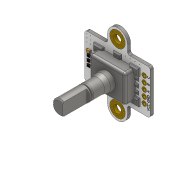
# Autodesk Inventor part: Rotary_Encoder_EC11
Saved by Autodesk Inventor 2017 (Build 210142000, 142)
## iProperties
Created: 2018-03-10
Part Number: Rotary_Encoder_EC11
Material: Generic
Document SubType Name: Modeling
Designer: Juan Carlos Botero
Density: 1 g/cm^3
Appearance: Stainless - Brushed
Author: Juan Carlos Botero
Autodesk Inventor part; units mm, degrees
ref_plane "YZ Plane" through (0, 0, 0) normal (1, 0, 0) x (0, 1, 0)
ref_plane "XZ Plane" through (0, 0, 0) normal (0, 1, 0) x (-1, 0, 0)
ref_plane "XY Plane" through (0, 0, 0) normal (0, 0, 1) x (1, 0, 0)
sketch "Sketch1" plane through (0, 0, 0) normal (0, 1, 0) x (-1, 0, 0)
  line L0 (13.715, 9.205) -> (13.715, -9.205)
  line L1 (-13.715, -9.205) -> (-13.715, 9.205)
  line L2 (-13.715, 9.205) -> (13.715, -9.205) construction
  line L3 (13.715, 9.205) -> (-13.715, -9.205) construction
  arc A0 (4.15, 12.7) -> (-4.15, 12.7) centre (0, 12.7) ccw
  arc A1 (-4.15, -12.7) -> (4.15, -12.7) centre (0, -12.7) ccw
  line L4 (0, 12.7) -> (0, -12.7) construction
  line L5 (4.15, 12.7) -> (4.15, 9.205)
  line L6 (4.15, -9.205) -> (4.15, -12.7)
  line L7 (-13.715, 9.205) -> (-4.15, 9.205)
  line L8 (4.15, 9.205) -> (13.715, 9.205)
  line L9 (13.715, -9.205) -> (4.15, -9.205)
  line L10 (-4.15, -9.205) -> (-13.715, -9.205)
  line L11 (-4.15, -12.7) -> (-4.15, -9.205)
  line L12 (-4.15, 9.205) -> (-4.15, 12.7)
  circle A2 centre (0, 12.7) radius 1.6
  circle A3 centre (0, -12.7) radius 1.6
  point P0 (0, 0)
  point P1 (0, 0)
  dimension "d0" = 27.43
  dimension "d1" = 18.41
  dimension "d2" = 25.4
  dimension "d3" = 8.3
  dimension "d4" = 3.2
  constraints: 26 end point, 5 parallel, 4 centre point, 4 midpoint, 4 point on circle, 4 tangent, 2 coincident, 2 equal radius, 2 horizontal, 2 perpendicular, 1 vertical
  measures "d0" distance of L0.end L1.start
  measures "d1" distance of L0.start L0.end
  measures "d2" distance of L4.start L4.end
  measures "d3" diameter of A1
  measures "d4" diameter of A2
extrude "Extrusion1" add sketch "Sketch1" along normal mid plane 1.32
fillet "Fillet1" radius 1 8 edges at (4.15, 0, 9.205) (-4.15, 0, 9.205) (-13.715, 0, 9.205) (-13.715, 0, -9.205) (-4.15, 0, -9.205) (4.15, 0, -9.205) (13.715, 0, -9.205) (13.715, 0, 9.205)
sketch "Sketch2" plane through (0, 0.66, 0) normal (0, 1, 0) x (1, 0, 0)
  arc A0 (12.715, -9.205) -> (13.715, -8.205) centre (12.715, -8.205) ccw projected
  line L0 (13.715, -8.205) -> (13.715, 8.205) projected
  arc A1 (13.715, 8.205) -> (12.715, 9.205) centre (12.715, 8.205) ccw projected
  line L1 (12.715, 9.205) -> (5.15, 9.205) projected
  arc A2 (4.15, 10.205) -> (5.15, 9.205) centre (5.15, 10.205) ccw projected
  line L2 (4.15, 10.205) -> (4.15, 12.7) projected
  arc A3 (4.15, 12.7) -> (-4.15, 12.7) centre (0, 12.7) ccw projected
  line L3 (-4.15, 12.7) -> (-4.15, 10.205) projected
  arc A4 (-5.15, 9.205) -> (-4.15, 10.205) centre (-5.15, 10.205) ccw projected
  line L4 (-5.15, 9.205) -> (-12.715, 9.205) projected
  arc A5 (-12.715, 9.205) -> (-13.715, 8.205) centre (-12.715, 8.205) ccw projected
  line L5 (-13.715, 8.205) -> (-13.715, -8.205) projected
  arc A6 (-13.715, -8.205) -> (-12.715, -9.205) centre (-12.715, -8.205) ccw projected
  line L6 (-12.715, -9.205) -> (-5.15, -9.205) projected
  arc A7 (-4.15, -10.205) -> (-5.15, -9.205) centre (-5.15, -10.205) ccw projected
  line L7 (-4.15, -10.205) -> (-4.15, -12.7) projected
  arc A8 (-4.15, -12.7) -> (4.15, -12.7) centre (0, -12.7) ccw projected
  line L8 (4.15, -12.7) -> (4.15, -10.205) projected
  arc A9 (5.15, -9.205) -> (4.15, -10.205) centre (5.15, -10.205) ccw projected
  line L9 (5.15, -9.205) -> (12.715, -9.205) projected
  circle A10 centre (0, 12.7) radius 1.6 projected
  circle A11 centre (0, -12.7) radius 1.6 projected
  circle A12 centre (0, -12.7) radius 3.25
  circle A13 centre (0, 12.7) radius 3.25
  point P0 (0, 0)
  dimension "d8" = 6.5
  dimension "d9" = 6.5
  constraints: 2 centre point, 2 coincident
  measures "d8" diameter of A12
  measures "d9" diameter of A13
extrude "Extrusion2" add sketch "Sketch2" along normal blind 0.01 contours A12 | A13
mirror "Mirror1" about plane through (0, 0, 0) normal (0, 1, 0) of "Extrusion2"
sketch "Sketch3" plane through (0, 0.67, -12.7) normal (0, 1, 0) x (1, 0, 0)
  circle A0 centre (0, -25.4) radius 1.6 projected
  circle A1 centre (0, -25.4) radius 3.25 projected
  circle A2 centre (-2.5, -25.4) radius 0.25
  circle A3 centre (0, -25.4) radius 2.5 construction
  point P0 (0, -12.7)
  dimension "d12" = 5
  dimension "d13" = 0.5
  constraints: 1 centre point, 1 coincident, 1 horizontal alignment, 2 other
  measures "d13" diameter of A2
extrude "Extrusion3" cut sketch "Sketch3" against normal through all contours A2
pattern_circular "Circular Pattern1" count 8 over 360 about axis through (0, 0, 12.7) along (0, 1, 0) of "Extrusion3"
sketch "Sketch4" plane through (0, 0.67, -12.7) normal (0, 1, 0) x (1, 0, 0)
  circle A0 centre (0, 0) radius 1.6 projected
  circle A1 centre (0, 0) radius 3.25 projected
  circle A2 centre (0, 0) radius 2.5 construction
  circle A3 centre (-2.5, 0) radius 0.25
  point P0 (0, -12.7)
  dimension "d19" = 5
  dimension "d20" = 0.5
  constraints: 1 centre point, 1 coincident, 1 horizontal alignment, 2 other
  measures "d20" diameter of A3
extrude "Extrusion4" cut sketch "Sketch4" against normal through all contours A3
pattern_circular "Circular Pattern2" count 8 over 360 about axis through (0, 0, -12.7) along (0, 1, 0) of "Extrusion4"
sketch "Sketch5" plane through (0, -0.66, 0) normal (0, -1, 0) x (1, 0, 0)
  line L0 (7.5, -6) -> (-7.5, -6)
  line L1 (-7.5, -6) -> (-7.5, 6)
  line L2 (-7.5, 6) -> (7.5, 6)
  line L3 (7.5, 6) -> (7.5, -6)
  line L4 (7.5, -6) -> (-7.5, 6) construction
  line L5 (-7.5, -6) -> (7.5, 6) construction
  point P0 (0, 0)
  dimension "d26" = 15
  dimension "d27" = 12
  constraints: 12 end point, 2 midpoint, 2 parallel, 1 horizontal, 1 perpendicular
  measures "d26" distance of L1.end L2.end
  measures "d27" distance of L0.end L1.end
extrude "Extrusion5" add sketch "Sketch5" along normal blind 4.4
sketch "Sketch6" plane through (0, -5.06, 0) normal (0, -1, 0) x (1, 0, 0)
  circle A0 centre (0, 0) radius 3.475
  dimension "d30" = 6.95
  constraints: 1 centre point, 1 coincident
  measures "d30" diameter of A0
extrude "Extrusion6" add sketch "Sketch6" along normal blind 2
sketch "Sketch7" plane through (0, -7.06, 0) normal (0, -1, 0) x (1, 0, 0)
  circle A0 centre (0, 0) radius 3.475 projected
extrude "Extrusion7" add sketch "Sketch7" along normal blind 2 draft -13
sketch "Sketch8" plane through (0, -9.06, 0) normal (0, -1, 0) x (1, 0, 0)
  circle A0 centre (0, 0) radius 3.0133 projected
extrude "Extrusion8" add sketch "Sketch8" along normal blind 5
fillet "Fillet2" radius 0.5 1 edges at (-3.0133, -14.06, 0)
sketch "Sketch9" plane through (0, -14.06, 0) normal (0, -1, 0) x (1, 0, 0)
  circle A0 centre (0, 0) radius 1.5
  dimension "d38" = 3
  constraints: 1 centre point, 1 coincident
  measures "d38" diameter of A0
extrude "Extrusion9" add sketch "Sketch9" along normal blind 0.5
sketch "Sketch10" plane through (0, -14.56, 0) normal (0, -1, 0) x (1, 0, 0)
  circle A0 centre (0, 0) radius 3.0133 projected
  circle A1 centre (0, 0) radius 3.0133 projected
extrude "Extrusion10" add sketch "Sketch10" along normal blind 10.5
chamfer "Chamfer1" distance 0.5 angle 45 1 edges at (-3.0133, -25.06, 0)
sketch "Sketch11" plane through (0, -25.06, 0) normal (0, -1, 0) x (1, 0, 0)
  line L0 (1.4867, 2.6209) -> (3.0133, 2.6209)
  line L1 (3.0133, 2.6209) -> (3.0133, -2.6209)
  line L2 (3.0133, -2.6209) -> (1.4867, -2.6209)
  line L3 (1.4867, -2.6209) -> (1.4867, 2.6209)
  circle A0 centre (0, 0) radius 3.0133 projected
  circle A1 centre (0, 0) radius 3.0133 projected
  line L4 (1.4867, 0) -> (-3.0133, 0)
  point P0 (3.0133, 0)
  dimension "d46" = 4.5
  constraints: 10 end point, 3 point on circle, 2 horizontal, 2 midpoint, 2 parallel, 1 horizontal alignment, 1 perpendicular, 1 point on line, 1 other
  measures "d46" distance of L4.start L4.end
extrude "Extrusion11" cut sketch "Sketch11" against normal blind 10 contours A0 L3 | L0 L1 A0 | L1 L2 A0
sketch "Sketch12" plane through (0, -0.66, 0) normal (0, -1, 0) x (1, 0, 0)
  circle A0 centre (11.215, -5.08) radius 0.5
  circle A1 centre (11.215, -2.54) radius 0.5
  circle A2 centre (11.215, 0) radius 0.5
  circle A3 centre (11.215, 2.54) radius 0.5
  circle A4 centre (11.215, 5.08) radius 0.5
  line L0 (13.715, -8.205) -> (13.715, 8.205) projected
  point P0 (0, 0)
  dimension "d49" = 2.54
  dimension "d50" = 2.54
  dimension "d51" = 2.54
  dimension "d52" = 2.54
  dimension "d53" = 1
  dimension "d54" = 2.5
  constraints: 5 centre point, 4 equal radius, 4 vertical alignment, 1 horizontal alignment
  measures "d49" distance of A1.centre A0.centre
  measures "d50" distance of A1.centre A2.centre
  measures "d51" distance of A2.centre A3.centre
  measures "d52" distance of A3.centre A4.centre
  measures "d53" diameter of A0
  measures "d54" distance from line of L0 A1.centre
extrude "Extrusion12" cut sketch "Sketch12" against normal through all
sketch "Sketch13" plane through (0, -0.66, 0) normal (0, -1, 0) x (1, 0, 0)
  circle A0 centre (11.215, 2.54) radius 0.5 projected
  circle A1 centre (11.215, -2.54) radius 0.5 projected
  circle A2 centre (11.215, -5.08) radius 0.5 projected
  circle A3 centre (11.215, 0) radius 0.5 projected
  circle A4 centre (11.215, 5.08) radius 0.5 projected
  line L0 (-7.5, -6) -> (-7.5, 6) projected
  line L1 (-7.5, 6) -> (7.5, 6) projected
  line L2 (7.5, 6) -> (7.5, -6) projected
  line L3 (7.5, -6) -> (-7.5, -6) projected
  circle A5 centre (0, 12.7) radius 3.25 projected
  circle A6 centre (0, -12.7) radius 3.25 projected
  arc A7 (13.715, 8.205) -> (12.715, 9.205) centre (12.715, 8.205) ccw projected
  line L4 (12.715, 9.205) -> (5.15, 9.205) projected
  arc A8 (4.15, 10.205) -> (5.15, 9.205) centre (5.15, 10.205) ccw projected
  line L5 (4.15, 10.205) -> (4.15, 12.7) projected
  arc A9 (4.15, 12.7) -> (-4.15, 12.7) centre (0, 12.7) ccw projected
  line L6 (-4.15, 12.7) -> (-4.15, 10.205) projected
  arc A10 (-5.15, 9.205) -> (-4.15, 10.205) centre (-5.15, 10.205) ccw projected
  line L7 (-5.15, 9.205) -> (-12.715, 9.205) projected
  arc A11 (-12.715, 9.205) -> (-13.715, 8.205) centre (-12.715, 8.205) ccw projected
  line L8 (-13.715, 8.205) -> (-13.715, -8.205) projected
  arc A12 (-13.715, -8.205) -> (-12.715, -9.205) centre (-12.715, -8.205) ccw projected
  line L9 (-12.715, -9.205) -> (-5.15, -9.205) projected
  arc A13 (-4.15, -10.205) -> (-5.15, -9.205) centre (-5.15, -10.205) ccw projected
  line L10 (-4.15, -10.205) -> (-4.15, -12.7) projected
  arc A14 (-4.15, -12.7) -> (4.15, -12.7) centre (0, -12.7) ccw projected
  line L11 (4.15, -12.7) -> (4.15, -10.205) projected
  arc A15 (5.15, -9.205) -> (4.15, -10.205) centre (5.15, -10.205) ccw projected
  line L12 (5.15, -9.205) -> (12.715, -9.205) projected
  arc A16 (12.715, -9.205) -> (13.715, -8.205) centre (12.715, -8.205) ccw projected
  line L13 (13.715, -8.205) -> (13.715, 8.205) projected
  circle A17 centre (11.215, -5.08) radius 1
  circle A18 centre (11.215, -2.54) radius 1
  circle A19 centre (11.215, 0) radius 1
  circle A20 centre (11.215, 2.54) radius 1
  circle A21 centre (11.215, 5.08) radius 1
  point P0 (0, 0)
  dimension "d57" = 0.5
  constraints: 5 centre point, 4 equal radius
  measures "d57" radial gap between concentric circles of A2 A17
extrude "Extrusion13" add sketch "Sketch13" along normal blind 0.01 contours A17 | A18 | A19 | A20 | A21
mirror "Mirror2" about plane through (0, 0, 0) normal (0, 1, 0) of "Extrusion13"
fillet "Fillet3" radius 1 8 edges at (0, -5.06, -6) (7.5, -5.06, 0) (7.5, -2.86, -6) (7.5, -2.86, 6) (0, -5.06, 6) (-7.5, -2.86, 6) (-7.5, -5.06, 0) (-7.5, -2.86, -6)
sketch "Sketch14" plane through (0, -0.66, 0) normal (0, -1, 0) x (1, 0, 0)
  line L0 (12.4092, -6.8272) -> (12.4092, 6.4026) construction
  line L1 (12.4092, 6.4026) -> (14.0609, 6.4026) construction
  line L2 (14.0609, 6.4026) -> (14.0609, -6.8272) construction
  line L3 (14.0609, -6.8272) -> (12.4092, -6.8272) construction
  line L4 (12.4271, -6.0006) -> (13.4271, -6.345)
  line L5 (13.4271, -6.345) -> (13.4271, -6.4885)
  line L6 (13.4271, -6.4885) -> (12.4271, -6.8329)
  line L7 (12.4271, -6.8329) -> (12.4271, -6.6903)
  line L8 (12.4271, -6.6903) -> (13.2577, -6.4131)
  line L9 (13.2577, -6.4131) -> (12.4271, -6.136)
  line L10 (12.4271, -6.136) -> (12.4271, -6.0006)
  spline S0 degree 2 poles (13.4449, -5.5144) (13.4449, -5.6117) (13.3793, -5.7762) (13.3136, -5.8361) knots 0 0 0 1 2 2 2
  spline S1 degree 2 poles (13.3136, -5.8361) (13.2488, -5.8961) (13.0543, -5.9617) (12.9279, -5.9617) knots 0 0 0 1 2 2 2
  spline S2 degree 2 poles (12.9279, -5.9617) (12.8023, -5.9617) (12.6159, -5.8977) (12.547, -5.8369) knots 0 0 0 1 2 2 2
  spline S3 degree 2 poles (12.547, -5.8369) (12.4797, -5.777) (12.4092, -5.6133) (12.4092, -5.512) knots 0 0 0 1 2 2 2
  spline S4 degree 2 poles (12.4092, -5.512) (12.4092, -5.4617) (12.4238, -5.3734) (12.4352, -5.3361) knots 0 0 0 1 2 2 2
  spline S5 degree 2 poles (12.4352, -5.3361) (12.4457, -5.3037) (12.4757, -5.2365) (12.4935, -5.2032) knots 0 0 0 1 2 2 2
  line L11 (12.4935, -5.2032) -> (12.654, -5.2032)
  line L12 (12.654, -5.2032) -> (12.654, -5.2138)
  spline S6 degree 2 poles (12.654, -5.2138) (12.6378, -5.2316) (12.5924, -5.2867) (12.5705, -5.3264) knots 0 0 0 1 2 2 2
  spline S7 degree 2 poles (12.5705, -5.3264) (12.5494, -5.3645) (12.5227, -5.4544) (12.5227, -5.5128) knots 0 0 0 1 2 2 2
  spline S8 degree 2 poles (12.5227, -5.5128) (12.5227, -5.5768) (12.5754, -5.6911) (12.6256, -5.734) knots 0 0 0 1 2 2 2
  spline S9 degree 2 poles (12.6256, -5.734) (12.6767, -5.7762) (12.8314, -5.8232) (12.9279, -5.8232) knots 0 0 0 1 2 2 2
  spline S10 degree 2 poles (12.9279, -5.8232) (13.0308, -5.8232) (13.1791, -5.7737) (13.2301, -5.7308) knots 0 0 0 1 2 2 2
  spline S11 degree 2 poles (13.2301, -5.7308) (13.2796, -5.6886) (13.3298, -5.576) (13.3298, -5.5128) knots 0 0 0 1 2 2 2
  spline S12 degree 2 poles (13.3298, -5.5128) (13.3298, -5.4553) (13.3015, -5.3572) (13.2804, -5.3191) knots 0 0 0 1 2 2 2
  spline S13 degree 2 poles (13.2804, -5.3191) (13.2593, -5.2827) (13.2156, -5.2284) (13.2002, -5.213) knots 0 0 0 1 2 2 2
  line L13 (13.2002, -5.213) -> (13.2002, -5.2032)
  line L14 (13.2002, -5.2032) -> (13.359, -5.2032)
  spline S14 degree 2 poles (13.359, -5.2032) (13.3744, -5.2365) (13.4028, -5.2948) (13.4157, -5.3361) knots 0 0 0 1 2 2 2
  spline S15 degree 2 poles (13.4157, -5.3361) (13.4303, -5.3799) (13.4449, -5.4544) (13.4449, -5.5144) knots 0 0 0 1 2 2 2
  spline S16 degree 2 poles (13.4449, -4.6886) (13.4449, -4.7859) (13.3793, -4.9504) (13.3136, -5.0104) knots 0 0 0 1 2 2 2
  spline S17 degree 2 poles (13.3136, -5.0104) (13.2488, -5.0703) (13.0543, -5.136) (12.9279, -5.136) knots 0 0 0 1 2 2 2
  spline S18 degree 2 poles (12.9279, -5.136) (12.8023, -5.136) (12.6159, -5.072) (12.547, -5.0112) knots 0 0 0 1 2 2 2
  spline S19 degree 2 poles (12.547, -5.0112) (12.4797, -4.9512) (12.4092, -4.7875) (12.4092, -4.6862) knots 0 0 0 1 2 2 2
  spline S20 degree 2 poles (12.4092, -4.6862) (12.4092, -4.636) (12.4238, -4.5476) (12.4352, -4.5104) knots 0 0 0 1 2 2 2
  spline S21 degree 2 poles (12.4352, -4.5104) (12.4457, -4.478) (12.4757, -4.4107) (12.4935, -4.3775) knots 0 0 0 1 2 2 2
  line L15 (12.4935, -4.3775) -> (12.654, -4.3775)
  line L16 (12.654, -4.3775) -> (12.654, -4.388)
  spline S22 degree 2 poles (12.654, -4.388) (12.6378, -4.4058) (12.5924, -4.4609) (12.5705, -4.5006) knots 0 0 0 1 2 2 2
  spline S23 degree 2 poles (12.5705, -4.5006) (12.5494, -4.5387) (12.5227, -4.6287) (12.5227, -4.687) knots 0 0 0 1 2 2 2
  spline S24 degree 2 poles (12.5227, -4.687) (12.5227, -4.751) (12.5754, -4.8653) (12.6256, -4.9083) knots 0 0 0 1 2 2 2
  spline S25 degree 2 poles (12.6256, -4.9083) (12.6767, -4.9504) (12.8314, -4.9974) (12.9279, -4.9974) knots 0 0 0 1 2 2 2
  spline S26 degree 2 poles (12.9279, -4.9974) (13.0308, -4.9974) (13.1791, -4.948) (13.2301, -4.905) knots 0 0 0 1 2 2 2
  spline S27 degree 2 poles (13.2301, -4.905) (13.2796, -4.8629) (13.3298, -4.7502) (13.3298, -4.687) knots 0 0 0 1 2 2 2
  spline S28 degree 2 poles (13.3298, -4.687) (13.3298, -4.6295) (13.3015, -4.5314) (13.2804, -4.4933) knots 0 0 0 1 2 2 2
  spline S29 degree 2 poles (13.2804, -4.4933) (13.2593, -4.4569) (13.2156, -4.4026) (13.2002, -4.3872) knots 0 0 0 1 2 2 2
  line L17 (13.2002, -4.3872) -> (13.2002, -4.3775)
  line L18 (13.2002, -4.3775) -> (13.359, -4.3775)
  spline S30 degree 2 poles (13.359, -4.3775) (13.3744, -4.4107) (13.4028, -4.469) (13.4157, -4.5104) knots 0 0 0 1 2 2 2
  spline S31 degree 2 poles (13.4157, -4.5104) (13.4303, -4.5541) (13.4449, -4.6287) (13.4449, -4.6886) knots 0 0 0 1 2 2 2
  spline S32 degree 2 poles (13.4465, -3.405) (13.4465, -3.5112) (13.3817, -3.687) (13.316, -3.7502) knots 0 0 0 1 2 2 2
  spline S33 degree 2 poles (13.316, -3.7502) (13.2496, -3.8134) (13.0535, -3.8807) (12.9263, -3.8807) knots 0 0 0 1 2 2 2
  spline S34 degree 2 poles (12.9263, -3.8807) (12.8055, -3.8807) (12.6143, -3.8126) (12.5462, -3.7494) knots 0 0 0 1 2 2 2
  spline S35 degree 2 poles (12.5462, -3.7494) (12.4806, -3.6886) (12.4092, -3.5104) (12.4092, -3.4042) knots 0 0 0 1 2 2 2
  spline S36 degree 2 poles (12.4092, -3.4042) (12.4092, -3.3532) (12.4238, -3.2608) (12.4368, -3.2186) knots 0 0 0 1 2 2 2
  spline S37 degree 2 poles (12.4368, -3.2186) (12.4465, -3.1846) (12.4822, -3.1019) (12.4951, -3.0768) knots 0 0 0 1 2 2 2
  line L19 (12.4951, -3.0768) -> (12.6556, -3.0768)
  line L20 (12.6556, -3.0768) -> (12.6556, -3.0882)
  spline S38 degree 2 poles (12.6556, -3.0882) (12.6337, -3.1133) (12.594, -3.166) (12.5713, -3.2146) knots 0 0 0 1 2 2 2
  spline S39 degree 2 poles (12.5713, -3.2146) (12.5511, -3.2551) (12.5243, -3.3596) (12.5243, -3.4196) knots 0 0 0 1 2 2 2
  spline S40 degree 2 poles (12.5243, -3.4196) (12.5243, -3.5638) (12.7415, -3.7421) (12.9222, -3.7421) knots 0 0 0 1 2 2 2
  spline S41 degree 2 poles (12.9222, -3.7421) (13.0227, -3.7421) (13.1734, -3.6951) (13.2253, -3.6506) knots 0 0 0 1 2 2 2
  spline S42 degree 2 poles (13.2253, -3.6506) (13.2771, -3.6076) (13.3314, -3.4861) (13.3314, -3.4099) knots 0 0 0 1 2 2 2
  spline S43 degree 2 poles (13.3314, -3.4099) (13.3314, -3.354) (13.3152, -3.2421) (13.299, -3.204) knots 0 0 0 1 2 2 2
  line L21 (13.299, -3.204) -> (13.0405, -3.204)
  line L22 (13.0405, -3.204) -> (13.0405, -3.4358)
  line L23 (13.0405, -3.4358) -> (12.9238, -3.4358)
  line L24 (12.9238, -3.4358) -> (12.9238, -3.0728)
  line L25 (12.9238, -3.0728) -> (13.3606, -3.0728)
  spline S44 degree 2 poles (13.3606, -3.0728) (13.372, -3.0979) (13.4068, -3.1838) (13.4173, -3.2203) knots 0 0 0 1 2 2 2
  spline S45 degree 2 poles (13.4173, -3.2203) (13.4319, -3.2697) (13.4465, -3.3491) (13.4465, -3.405) knots 0 0 0 1 2 2 2
  line L26 (13.4271, -2.1903) -> (13.4271, -2.3394)
  line L27 (13.4271, -2.3394) -> (12.5648, -2.7818)
  line L28 (12.5648, -2.7818) -> (13.4271, -2.7818)
  line L29 (13.4271, -2.7818) -> (13.4271, -2.9058)
  line L30 (13.4271, -2.9058) -> (12.4271, -2.9058)
  line L31 (12.4271, -2.9058) -> (12.4271, -2.717)
  line L32 (12.4271, -2.717) -> (13.2188, -2.3143)
  line L33 (13.2188, -2.3143) -> (12.4271, -2.3143)
  line L34 (12.4271, -2.3143) -> (12.4271, -2.1903)
  line L35 (12.4271, -2.1903) -> (13.4271, -2.1903)
  spline S46 degree 2 poles (12.9279, -1.1992) (13.0648, -1.1992) (13.2853, -1.3102) (13.3468, -1.4034) knots 0 0 0 1 2 2 2
  spline S47 degree 2 poles (13.3468, -1.4034) (13.3947, -1.4796) (13.4271, -1.636) (13.4271, -1.7575) knots 0 0 0 1 2 2 2
  line L36 (13.4271, -1.7575) -> (13.4271, -1.9877)
  line L37 (13.4271, -1.9877) -> (12.4271, -1.9877)
  line L38 (12.4271, -1.9877) -> (12.4271, -1.76)
  spline S48 degree 2 poles (12.4271, -1.76) (12.4271, -1.619) (12.4692, -1.4585) (12.5065, -1.4018) knots 0 0 0 1 2 2 2
  spline S49 degree 2 poles (12.5065, -1.4018) (12.5705, -1.3053) (12.782, -1.1992) (12.9279, -1.1992) knots 0 0 0 1 2 2 2
  spline S50 degree 2 poles (12.9263, -1.3378) (12.8112, -1.3378) (12.6483, -1.4139) (12.6021, -1.4893) knots 0 0 0 1 2 2 2
  spline S51 degree 2 poles (12.6021, -1.4893) (12.5705, -1.5428) (12.5421, -1.6635) (12.5421, -1.7535) knots 0 0 0 1 2 2 2
  line L39 (12.5421, -1.7535) -> (12.5421, -1.8548)
  line L40 (12.5421, -1.8548) -> (13.312, -1.8548)
  line L41 (13.312, -1.8548) -> (13.312, -1.7535)
  spline S52 degree 2 poles (13.312, -1.7535) (13.312, -1.6651) (13.2836, -1.5314) (13.2455, -1.4771) knots 0 0 0 1 2 2 2
  spline S53 degree 2 poles (13.2455, -1.4771) (13.1985, -1.4074) (13.043, -1.3378) (12.9263, -1.3378) knots 0 0 0 1 2 2 2
  line L42 (13.4271, -0.3037) -> (12.4271, 0.0334)
  line L43 (12.4271, 0.0334) -> (12.4271, 0.1971)
  line L44 (12.4271, 0.1971) -> (13.4271, 0.5342)
  line L45 (13.4271, 0.5342) -> (13.4271, 0.394)
  line L46 (13.4271, 0.394) -> (13.1475, 0.3032)
  line L47 (13.1475, 0.3032) -> (13.1475, -0.0784)
  line L48 (13.1475, -0.0784) -> (13.4271, -0.1692)
  line L49 (13.4271, -0.1692) -> (13.4271, -0.3037)
  line L50 (13.034, 0.2668) -> (12.5632, 0.112)
  line L51 (12.5632, 0.112) -> (13.034, -0.042)
  line L52 (13.034, -0.042) -> (13.034, 0.2668)
  spline S54 degree 2 poles (13.1199, 3.0253) (13.1945, 3.0253) (13.3088, 2.9686) (13.346, 2.9216) knots 0 0 0 1 2 2 2
  spline S55 degree 2 poles (13.346, 2.9216) (13.3898, 2.8648) (13.4271, 2.736) (13.4271, 2.6339) knots 0 0 0 1 2 2 2
  line L53 (13.4271, 2.6339) -> (13.4271, 2.347)
  line L54 (13.4271, 2.347) -> (12.4271, 2.347)
  line L55 (12.4271, 2.347) -> (12.4271, 2.612)
  spline S56 degree 2 poles (12.4271, 2.612) (12.4271, 2.719) (12.4408, 2.8259) (12.4676, 2.8746) knots 0 0 0 1 2 2 2
  spline S57 degree 2 poles (12.4676, 2.8746) (12.4959, 2.9289) (12.5891, 2.9783) (12.6524, 2.9783) knots 0 0 0 1 2 2 2
  spline S58 degree 2 poles (12.6524, 2.9783) (12.7229, 2.9783) (12.8347, 2.9037) (12.8663, 2.8381) knots 0 0 0 1 2 2 2
  line L56 (12.8663, 2.8381) -> (12.8712, 2.8381)
  spline S59 degree 2 poles (12.8712, 2.8381) (12.8955, 2.9272) (13.0243, 3.0253) (13.1199, 3.0253) knots 0 0 0 1 2 2 2
  spline S60 degree 2 poles (13.1256, 2.8867) (13.0689, 2.8867) (12.9959, 2.8543) (12.97, 2.8057) knots 0 0 0 1 2 2 2
  spline S61 degree 2 poles (12.97, 2.8057) (12.9538, 2.7741) (12.9441, 2.6995) (12.9441, 2.6306) knots 0 0 0 1 2 2 2
  line L57 (12.9441, 2.6306) -> (12.9441, 2.4799)
  line L58 (12.9441, 2.4799) -> (13.3136, 2.4799)
  line L59 (13.3136, 2.4799) -> (13.3136, 2.5877)
  spline S62 degree 2 poles (13.3136, 2.5877) (13.3136, 2.6752) (13.2974, 2.7757) (13.2715, 2.8146) knots 0 0 0 1 2 2 2
  spline S63 degree 2 poles (13.2715, 2.8146) (13.2447, 2.8519) (13.1783, 2.8867) (13.1256, 2.8867) knots 0 0 0 1 2 2 2
  spline S64 degree 2 poles (12.671, 2.8397) (12.6353, 2.8397) (12.5818, 2.8154) (12.5665, 2.7887) knots 0 0 0 1 2 2 2
  spline S65 degree 2 poles (12.5665, 2.7887) (12.5486, 2.7562) (12.5405, 2.6776) (12.5405, 2.6071) knots 0 0 0 1 2 2 2
  line L60 (12.5405, 2.6071) -> (12.5405, 2.4799)
  line L61 (12.5405, 2.4799) -> (12.8331, 2.4799)
  line L62 (12.8331, 2.4799) -> (12.8331, 2.6306)
  spline S66 degree 2 poles (12.8331, 2.6306) (12.8331, 2.693) (12.8201, 2.7522) (12.7998, 2.7838) knots 0 0 0 1 2 2 2
  spline S67 degree 2 poles (12.7998, 2.7838) (12.7804, 2.8146) (12.718, 2.8397) (12.671, 2.8397) knots 0 0 0 1 2 2 2
  spline S68 degree 2 poles (13.4449, 5.266) (13.4449, 5.1687) (13.3793, 5.0042) (13.3136, 4.9443) knots 0 0 0 1 2 2 2
  spline S69 degree 2 poles (13.3136, 4.9443) (13.2488, 4.8843) (13.0543, 4.8186) (12.9279, 4.8186) knots 0 0 0 1 2 2 2
  spline S70 degree 2 poles (12.9279, 4.8186) (12.8023, 4.8186) (12.6159, 4.8827) (12.547, 4.9434) knots 0 0 0 1 2 2 2
  spline S71 degree 2 poles (12.547, 4.9434) (12.4797, 5.0034) (12.4092, 5.1671) (12.4092, 5.2684) knots 0 0 0 1 2 2 2
  spline S72 degree 2 poles (12.4092, 5.2684) (12.4092, 5.3186) (12.4238, 5.407) (12.4352, 5.4443) knots 0 0 0 1 2 2 2
  spline S73 degree 2 poles (12.4352, 5.4443) (12.4457, 5.4767) (12.4757, 5.5439) (12.4935, 5.5772) knots 0 0 0 1 2 2 2
  line L63 (12.4935, 5.5772) -> (12.654, 5.5772)
  line L64 (12.654, 5.5772) -> (12.654, 5.5666)
  spline S74 degree 2 poles (12.654, 5.5666) (12.6378, 5.5488) (12.5924, 5.4937) (12.5705, 5.454) knots 0 0 0 1 2 2 2
  spline S75 degree 2 poles (12.5705, 5.454) (12.5494, 5.4159) (12.5227, 5.3259) (12.5227, 5.2676) knots 0 0 0 1 2 2 2
  spline S76 degree 2 poles (12.5227, 5.2676) (12.5227, 5.2036) (12.5754, 5.0893) (12.6256, 5.0464) knots 0 0 0 1 2 2 2
  spline S77 degree 2 poles (12.6256, 5.0464) (12.6767, 5.0042) (12.8314, 4.9572) (12.9279, 4.9572) knots 0 0 0 1 2 2 2
  spline S78 degree 2 poles (12.9279, 4.9572) (13.0308, 4.9572) (13.1791, 5.0067) (13.2301, 5.0496) knots 0 0 0 1 2 2 2
  spline S79 degree 2 poles (13.2301, 5.0496) (13.2796, 5.0917) (13.3298, 5.2044) (13.3298, 5.2676) knots 0 0 0 1 2 2 2
  spline S80 degree 2 poles (13.3298, 5.2676) (13.3298, 5.3251) (13.3015, 5.4232) (13.2804, 5.4613) knots 0 0 0 1 2 2 2
  spline S81 degree 2 poles (13.2804, 5.4613) (13.2593, 5.4977) (13.2156, 5.552) (13.2002, 5.5674) knots 0 0 0 1 2 2 2
  line L65 (13.2002, 5.5674) -> (13.2002, 5.5772)
  line L66 (13.2002, 5.5772) -> (13.359, 5.5772)
  spline S82 degree 2 poles (13.359, 5.5772) (13.3744, 5.5439) (13.4028, 5.4856) (13.4157, 5.4443) knots 0 0 0 1 2 2 2
  spline S83 degree 2 poles (13.4157, 5.4443) (13.4303, 5.4005) (13.4449, 5.3259) (13.4449, 5.266) knots 0 0 0 1 2 2 2
  point P0 (0, 0)
  constraints: 2 other
extrude "Extrusion14" add sketch "Sketch14" along normal blind 0.01
sketch "Sketch15" plane through (0, -0.66, 0) normal (0, -1, 0) x (1, 0, 0)
  line L0 (-1.75, 5.5) -> (1.75, 5.5)
  line L1 (1.75, 5.5) -> (1.75, 8)
  line L2 (1.75, 8) -> (-1.75, 8)
  line L3 (-1.75, 8) -> (-1.75, 5.5)
  line L4 (-1.75, 5.5) -> (1.75, 8) construction
  line L5 (1.75, 5.5) -> (-1.75, 8) construction
  line L6 (-1.75, -8) -> (1.75, -8)
  line L7 (1.75, -8) -> (1.75, -5.5)
  line L8 (1.75, -5.5) -> (-1.75, -5.5)
  line L9 (-1.75, -5.5) -> (-1.75, -8)
  line L10 (-1.75, -8) -> (1.75, -5.5) construction
  line L11 (1.75, -8) -> (-1.75, -5.5) construction
  line L12 (0, 6.75) -> (0, -6.75) construction
  line L13 (7, 1.75) -> (9, 1.75)
  line L14 (9, 1.75) -> (9, 3.25)
  line L15 (9, 3.25) -> (7, 3.25)
  line L16 (7, 3.25) -> (7, 1.75)
  line L17 (7, 1.75) -> (9, 3.25) construction
  line L18 (9, 1.75) -> (7, 3.25) construction
  line L19 (7, -0.75) -> (9, -0.75)
  line L20 (9, -0.75) -> (9, 0.75)
  line L21 (9, 0.75) -> (7, 0.75)
  line L22 (7, 0.75) -> (7, -0.75)
  line L23 (7, -0.75) -> (9, 0.75) construction
  line L24 (9, -0.75) -> (7, 0.75) construction
  line L25 (7, -3.25) -> (9, -3.25)
  line L26 (9, -3.25) -> (9, -1.75)
  line L27 (9, -1.75) -> (7, -1.75)
  line L28 (7, -1.75) -> (7, -3.25)
  line L29 (7, -3.25) -> (9, -1.75) construction
  line L30 (9, -3.25) -> (7, -1.75) construction
  line L31 (8, -2.5) -> (8, 2.5) construction
  line L32 (-9, 1.75) -> (-7, 1.75)
  line L33 (-7, 1.75) -> (-7, 3.25)
  line L34 (-7, 3.25) -> (-9, 3.25)
  line L35 (-9, 3.25) -> (-9, 1.75)
  line L36 (-9, 1.75) -> (-7, 3.25) construction
  line L37 (-7, 1.75) -> (-9, 3.25) construction
  line L38 (-9, -3.25) -> (-7, -3.25)
  line L39 (-7, -3.25) -> (-7, -1.75)
  line L40 (-7, -1.75) -> (-9, -1.75)
  line L41 (-9, -1.75) -> (-9, -3.25)
  line L42 (-9, -3.25) -> (-7, -1.75) construction
  line L43 (-7, -3.25) -> (-9, -1.75) construction
  line L44 (-8, 2.5) -> (8, -2.5) construction
  line L45 (-8, -2.5) -> (8, 2.5) construction
  point P0 (0, 0)
  point P1 (0, 0)
  point P2 (8, 2.5)
  point P3 (8, 0)
  point P4 (8, -2.5)
  point P5 (8, 2.5)
  point P6 (8, 0)
  point P7 (8, 0)
  point P8 (0, 0)
  dimension "d63" = 2.5
  dimension "d64" = 3.5
  dimension "d65" = 16
  dimension "d67" = 2
  dimension "d68" = 1.5
  dimension "d69" = 6.5
  dimension "d72" = 6.5
  dimension "d73" = 18
  constraints: 92 end point, 23 midpoint, 14 parallel, 11 equal length, 7 horizontal, 7 perpendicular, 3 point on line, 3 vertical alignment, 2 vertical, 1 coincident, 1 horizontal alignment
  measures "d63" distance of L2.end L0.start
  measures "d64" distance of L1.end L2.end
  measures "d65" distance between parallel lines of L6 L2
  measures "d67" distance of L14.end L15.end
  measures "d68" distance of L13.end L14.end
  measures "d69" distance between parallel lines of L25 L15
  measures "d72" distance between parallel lines of L38 L34
  measures "d73" distance between parallel lines of L26 L41
extrude "Extrusion15" add sketch "Sketch15" along normal blind 0.5
sketch "Sketch16" plane through (0, -0.66, 0) normal (0, -1, 0) x (1, 0, 0)
  line L0 (-9.5, 4) -> (-5.5, 4)
  line L1 (-5.5, 4) -> (-5.5, 7)
  line L2 (-5.5, 7) -> (-9.5, 7)
  line L3 (-9.5, 7) -> (-9.5, 4)
  line L4 (-9.5, 4) -> (-5.5, 7) construction
  line L5 (-5.5, 4) -> (-9.5, 7) construction
  line L6 (5.5, 4) -> (9.5, 4)
  line L7 (9.5, 4) -> (9.5, 7)
  line L8 (9.5, 7) -> (5.5, 7)
  line L9 (5.5, 7) -> (5.5, 4)
  line L10 (5.5, 4) -> (9.5, 7) construction
  line L11 (9.5, 4) -> (5.5, 7) construction
  line L12 (5.5, -7) -> (9.5, -7)
  line L13 (9.5, -7) -> (9.5, -4)
  line L14 (9.5, -4) -> (5.5, -4)
  line L15 (5.5, -4) -> (5.5, -7)
  line L16 (5.5, -7) -> (9.5, -4) construction
  line L17 (9.5, -7) -> (5.5, -4) construction
  line L18 (-9.5, -7) -> (-5.5, -7)
  line L19 (-5.5, -7) -> (-5.5, -4)
  line L20 (-5.5, -4) -> (-9.5, -4)
  line L21 (-9.5, -4) -> (-9.5, -7)
  line L22 (-9.5, -7) -> (-5.5, -4) construction
  line L23 (-5.5, -7) -> (-9.5, -4) construction
  line L24 (6.5, 6) -> (-6.5, 6) projected
  line L25 (-6.5, -6) -> (6.5, -6) projected
  line L26 (-7.5, 5) -> (-7.5, -5) projected
  line L27 (7.5, -5) -> (7.5, 5) projected
  point P0 (0, 0)
  point P1 (-7.5, 5.5)
  point P2 (7.5, 5.5)
  point P3 (7.5, -5.5)
  point P4 (-7.5, -5.5)
  point P5 (-7.5, 5.5)
  point P6 (7.5, 5.5)
  point P7 (-7.5, -5.5)
  point P8 (7.5, -5.5)
  point P9 (-7.5, 5.5)
  point P10 (-7.5, -5.5)
  point P11 (7.5, 5.5)
  point P12 (7.5, -5.5)
  dimension "d76" = 1
  dimension "d77" = 1
  dimension "d78" = 3
  dimension "d79" = 4
  dimension "d80" = 2
  dimension "d81" = 2
  constraints: 48 end point, 16 midpoint, 8 parallel, 6 equal length, 4 horizontal, 4 perpendicular, 2 horizontal alignment, 2 vertical alignment, 1 point on line
  measures "d76" distance between parallel lines of L24 L2
  measures "d77" distance between parallel lines of L25 L18
  measures "d78" distance of L2.end L0.start
  measures "d79" distance of L1.end L2.end
  measures "d80" distance between parallel lines of L3 L26
  measures "d81" distance between parallel lines of L7 L27
extrude "Extrusion16" add sketch "Sketch16" along normal blind 1 contours L3 L2 L1 L0 | L20 L19 L18 L21 | L9 L8 L7 L6 | L15 L14 L13 L12
sketch "Sketch17" plane through (0, -0.66, 0) normal (0, -1, 0) x (1, 0, 0)
  circle A0 centre (0, 2.5) radius 0.5
  circle A1 centre (0, -2) radius 0.6
  point P0 (0, 0)
  dimension "d84" = 1
  dimension "d85" = 1.2
  dimension "d86" = 2.5
  dimension "d87" = 2
  constraints: 2 centre point, 2 vertical alignment
  measures "d84" diameter of A0
  measures "d85" diameter of A1
  measures "d86" distance of point (0, 0) A0.centre
  measures "d87" distance of A1.centre point (0, 0)
extrude "Extrusion17" cut sketch "Sketch17" against normal through all
sketch "Sketch18" plane through (0, -0.66, -2) normal (0, 1, 0) x (1, 0, 0)
  circle A0 centre (0, -4.5) radius 0.5 projected
  circle A1 centre (0, 0) radius 0.6 projected
  circle A2 centre (11.215, -7.08) radius 1 projected
  circle A3 centre (11.215, -2) radius 1 projected
  circle A4 centre (11.215, 3.08) radius 1 projected
  circle A5 centre (11.215, 0.54) radius 1 projected
  circle A6 centre (11.215, -4.54) radius 1 projected
  circle A7 centre (0, -14.7) radius 3.25 projected
  circle A8 centre (0, 10.7) radius 3.25 projected
  arc A9 (12.715, -11.205) -> (13.715, -10.205) centre (12.715, -10.205) ccw projected
  line L0 (13.715, -10.205) -> (13.715, 6.205) projected
  arc A10 (13.715, 6.205) -> (12.715, 7.205) centre (12.715, 6.205) ccw projected
  line L1 (12.715, 7.205) -> (5.15, 7.205) projected
  arc A11 (4.15, 8.205) -> (5.15, 7.205) centre (5.15, 8.205) ccw projected
  line L2 (4.15, 8.205) -> (4.15, 10.7) projected
  arc A12 (4.15, 10.7) -> (-4.15, 10.7) centre (0, 10.7) ccw projected
  line L3 (-4.15, 10.7) -> (-4.15, 8.205) projected
  arc A13 (-5.15, 7.205) -> (-4.15, 8.205) centre (-5.15, 8.205) ccw projected
  line L4 (-5.15, 7.205) -> (-12.715, 7.205) projected
  arc A14 (-12.715, 7.205) -> (-13.715, 6.205) centre (-12.715, 6.205) ccw projected
  line L5 (-13.715, 6.205) -> (-13.715, -10.205) projected
  arc A15 (-13.715, -10.205) -> (-12.715, -11.205) centre (-12.715, -10.205) ccw projected
  line L6 (-12.715, -11.205) -> (-5.15, -11.205) projected
  arc A16 (-4.15, -12.205) -> (-5.15, -11.205) centre (-5.15, -12.205) ccw projected
  line L7 (-4.15, -12.205) -> (-4.15, -14.7) projected
  arc A17 (-4.15, -14.7) -> (4.15, -14.7) centre (0, -14.7) ccw projected
  line L8 (4.15, -14.7) -> (4.15, -12.205) projected
  arc A18 (5.15, -11.205) -> (4.15, -12.205) centre (5.15, -12.205) ccw projected
  line L9 (5.15, -11.205) -> (12.715, -11.205) projected
  circle A19 centre (0, 0) radius 0.5
  circle A20 centre (0, -4.5) radius 0.4
  point P0 (0, -2)
  dimension "d45" = 45
  dimension "d90" = 0.1
  dimension "d91" = 0.1
  constraints: 2 centre point
  measures "d90" radial gap between concentric circles of A1 A19
  measures "d91" radial gap between concentric circles of A0 A20
extrude "Extrusion18" add sketch "Sketch18" along normal up to surface (1.32 mm away) contours A19 | A20
fillet "Fillet4" radius 0.2 2 edges at (-0.5, 0.66, -2) (-0.4, 0.66, 2.5)
chamfer "Chamfer2" distance 0.5 angle 45 37 edges at (-9.5, -1.66, -5.5) (-9, -1.16, -2.5) (-9, -1.16, 2.5) (0, -1.16, -8) (0, -1.16, 8) (1.75, -1.16, 7) (-1.75, -1.16, 7) (1.75, -1.16, -7) (-1.75, -1.16, -7) (8.25, -1.16, -3.25) (9, -1.16, -2.5) (8.25, -1.16, -1.75) (8.25, -1.16, -0.75) (9, -1.16, 0) (8.25, -1.16, 0.75) (8.25, -1.16, 1.75) (9, -1.16, 2.5) (8.25, -1.16, 3.25) (-8.25, -1.16, -3.25) (-8.25, -1.16, -1.75) (-8.25, -1.16, 1.75) (-8.25, -1.16, 3.25) (-7.5, -1.66, -7) (7.5, -1.66, -7) (9.5, -1.66, -5.5) (9.5, -1.66, 5.5) (7.5, -1.66, 7) (-7.5, -1.66, 7) (-9.5, -1.66, 5.5) (-5.5, -1.66, 6.5) (8.5, -1.66, 4) (8.5, -1.66, -4) (5.5, -1.66, 6.5) (-8.5, -1.66, -4) (-8.5, -1.66, 4) (-5.5, -1.66, -6.5) (5.5, -1.66, -6.5)
sketch "Sketch19" plane through (0, -0.66, 0) normal (0, -1, 0) x (1, 0, 0)
  line L0 (-10.865, -3.2) -> (-12.565, -3.2)
  line L1 (-12.565, -3.2) -> (-12.565, -2.2)
  line L2 (-12.565, -2.2) -> (-10.865, -2.2)
  line L3 (-10.865, -2.2) -> (-10.865, -3.2)
  line L4 (-10.865, -3.2) -> (-12.565, -2.2) construction
  line L5 (-12.565, -3.2) -> (-10.865, -2.2) construction
  line L6 (-10.865, -1.4) -> (-12.565, -1.4)
  line L7 (-12.565, -1.4) -> (-12.565, -0.4)
  line L8 (-12.565, -0.4) -> (-10.865, -0.4)
  line L9 (-10.865, -0.4) -> (-10.865, -1.4)
  line L10 (-10.865, -1.4) -> (-12.565, -0.4) construction
  line L11 (-12.565, -1.4) -> (-10.865, -0.4) construction
  line L12 (-10.865, 0.4) -> (-12.565, 0.4)
  line L13 (-12.565, 0.4) -> (-12.565, 1.4)
  line L14 (-12.565, 1.4) -> (-10.865, 1.4)
  line L15 (-10.865, 1.4) -> (-10.865, 0.4)
  line L16 (-10.865, 0.4) -> (-12.565, 1.4) construction
  line L17 (-12.565, 0.4) -> (-10.865, 1.4) construction
  line L18 (-10.865, 2.2) -> (-12.565, 2.2)
  line L19 (-12.565, 2.2) -> (-12.565, 3.2)
  line L20 (-12.565, 3.2) -> (-10.865, 3.2)
  line L21 (-10.865, 3.2) -> (-10.865, 2.2)
  line L22 (-10.865, 2.2) -> (-12.565, 3.2) construction
  line L23 (-12.565, 2.2) -> (-10.865, 3.2) construction
  line L24 (-13.715, 8.205) -> (-13.715, -8.205) projected
  line L25 (-11.715, -0.9) -> (-11.715, 0.9) construction
  point P0 (0, 0)
  point P1 (-11.715, -2.7)
  point P2 (-11.715, -0.9)
  point P3 (-11.715, 0.9)
  point P4 (-11.715, 2.7)
  point P5 (-11.715, -2.7)
  point P6 (-11.715, -0.9)
  point P7 (-11.715, 0.9)
  point P8 (-11.715, 2.7)
  point P9 (-11.715, 0)
  dimension "d98" = 1
  dimension "d99" = 2
  dimension "d100" = 1.7
  dimension "d101" = 1.8
  dimension "d102" = 1.8
  dimension "d103" = 1.8
  constraints: 50 end point, 15 midpoint, 8 parallel, 6 equal length, 4 horizontal, 4 perpendicular, 3 vertical alignment, 1 horizontal alignment, 1 point on line, 1 vertical
  measures "d98" distance of L0.end L1.end
  measures "d99" distance from line of L24 point (-11.715, -2.7)
  measures "d100" distance of L0.start L0.end
  measures "d101" distance of point (-11.715, -0.9) point (-11.715, -2.7)
  measures "d102" distance of L25.end point (-11.715, -0.9)
  measures "d103" distance of point (-11.715, 0.9) point (-11.715, 2.7)
extrude "Extrusion19" add sketch "Sketch19" along normal blind 0.5 contours L0 L1 L2 L3 | L6 L7 L8 L9 | L12 L13 L14 L15
extrude "Extrusion21" add sketch "Sketch19" along normal blind 0.8 contours L18 L19 L20 L21
fillet "Fillet5" radius 0.2 16 edges at (-12.565, -1.16, -2.7) (-11.715, -1.16, -2.2) (-11.715, -1.16, -3.2) (-10.865, -1.16, -2.7) (-11.715, -1.16, -1.4) (-11.715, -1.16, -0.4) (-12.565, -1.16, -0.9) (-10.865, -1.16, -0.9) (-10.865, -1.16, 0.9) (-11.715, -1.16, 0.4) (-11.715, -1.16, 1.4) (-12.565, -1.16, 0.9) (-11.715, -1.46, 2.2) (-12.565, -1.46, 2.7) (-10.865, -1.46, 2.7) (-11.715, -1.46, 3.2)
sketch "Sketch20" plane through (0, -0.66, 0) normal (0, -1, 0) x (1, 0, 0)
  line L0 (-11.065, -2.4) -> (-11.065, -3) projected
  line L1 (-12.365, -2.4) -> (-11.065, -2.4) projected
  line L2 (-12.365, -3) -> (-12.365, -2.4) projected
  line L3 (-11.065, -3) -> (-12.365, -3) projected
  line L4 (-12.365, -0.6) -> (-11.065, -0.6) projected
  line L5 (-12.365, -1.2) -> (-12.365, -0.6) projected
  line L6 (-11.065, -1.2) -> (-12.365, -1.2) projected
  line L7 (-11.065, -0.6) -> (-11.065, -1.2) projected
  line L8 (-12.365, 0.6) -> (-12.365, 1.2) projected
  line L9 (-11.065, 0.6) -> (-12.365, 0.6) projected
  line L10 (-11.065, 1.2) -> (-11.065, 0.6) projected
  line L11 (-12.365, 1.2) -> (-11.065, 1.2) projected
  line L12 (-12.365, 2.4) -> (-12.365, 3) projected
  line L13 (-11.065, 2.4) -> (-12.365, 2.4) projected
  line L14 (-11.065, 3) -> (-11.065, 2.4) projected
  line L15 (-12.365, 3) -> (-11.065, 3) projected
  line L16 (-11.065, -3.21) -> (-12.365, -3.21)
  line L17 (-12.365, -3.21) -> (-12.365, -2.19)
  line L18 (-12.365, -2.19) -> (-11.065, -2.19)
  line L19 (-11.065, -2.19) -> (-11.065, -3.21)
  line L20 (-11.065, -3.21) -> (-12.365, -2.19) construction
  line L21 (-12.365, -3.21) -> (-11.065, -2.19) construction
  line L22 (-11.065, -1.41) -> (-12.365, -1.41)
  line L23 (-12.365, -1.41) -> (-12.365, -0.39)
  line L24 (-12.365, -0.39) -> (-11.065, -0.39)
  line L25 (-11.065, -0.39) -> (-11.065, -1.41)
  line L26 (-11.065, -1.41) -> (-12.365, -0.39) construction
  line L27 (-12.365, -1.41) -> (-11.065, -0.39) construction
  line L28 (-11.065, 1.41) -> (-12.365, 1.41)
  line L29 (-12.365, 1.41) -> (-12.365, 0.39)
  line L30 (-12.365, 0.39) -> (-11.065, 0.39)
  line L31 (-11.065, 0.39) -> (-11.065, 1.41)
  line L32 (-11.065, 1.41) -> (-12.365, 0.39) construction
  line L33 (-12.365, 1.41) -> (-11.065, 0.39) construction
  line L34 (-11.065, 3.21) -> (-12.365, 3.21)
  line L35 (-12.365, 3.21) -> (-12.365, 2.19)
  line L36 (-12.365, 2.19) -> (-11.065, 2.19)
  line L37 (-11.065, 2.19) -> (-11.065, 3.21)
  line L38 (-11.065, 3.21) -> (-12.365, 2.19) construction
  line L39 (-12.365, 3.21) -> (-11.065, 2.19) construction
  line L40 (-10.865, -2.2) -> (-12.565, -2.2) projected
  line L41 (-12.565, -3.2) -> (-10.865, -3.2) projected
  point P0 (0, 0)
  point P1 (-11.715, -2.7)
  point P2 (-11.715, -0.9)
  point P3 (-11.715, 0.9)
  point P4 (-11.715, 2.7)
  dimension "d112" = 0.01
  dimension "d113" = 0.01
  constraints: 48 end point, 8 midpoint, 8 parallel, 6 equal length, 4 horizontal, 4 perpendicular, 3 point on line
  measures "d112" distance between parallel lines of L18 L40
  measures "d113" distance between parallel lines of L41 L16
extrude "Extrusion20" add sketch "Sketch20" along normal blind 0.5 contours L0 L3 L2 L1 | L1 L17 L40 L19 | L19 L41 L17 L3 | L40 L17 L18 L19 | L19 L16 L17 L41 | L23 L24 L25 L4 | L4 L7 L6 L5 | L6 L25 L22 L23 | L8 L11 L10 L9 | L9 L31 L30 L29 | L29 L28 L31 L11
extrude "Extrusion22" add sketch "Sketch20" along normal blind 0.8 contours L12 L15 L14 L13 | L13 L37 L36 L35 | L35 L34 L37 L15
fillet "Fillet6" radius 0.1 8 edges at (-11.715, -1.16, -1.41) (-11.715, -1.16, -0.39) (-11.715, -1.16, -2.19) (-11.715, -1.16, -3.21) (-11.715, -1.16, 0.39) (-11.715, -1.16, 1.41) (-11.715, -1.46, 2.19) (-11.715, -1.46, 3.21)
fillet "Fillet7" radius 0.1 2 edges at (-0.6, 0.66, -2) (-0.5, 0.66, 2.5)
sketch "Sketch21" plane through (0, -0.66, 0) normal (0, -1, 0) x (1, 0, 0)
  circle A0 centre (-12.8407, 8.2123) radius 0.1
  point P0 (0, 0)
  dimension "d120" = 0.2
  constraints: 1 centre point
  measures "d120" diameter of A0
extrude "Extrusion23" cut sketch "Sketch21" against normal through all
pattern_linear "Rectangular Pattern1" count 3 spacing 1.5 along (0, 0, -1) count 2 spacing 1.5 along (1, 0, 0) of "Extrusion23" second direction both ways yes
sketch "Sketch22" plane through (0, -0.66, 0) normal (0, -1, 0) x (1, 0, 0)
  circle A0 centre (9.3, 8.205) radius 0.1
  line L0 (12.715, 9.205) -> (5.15, 9.205) projected
  line L1 (9.5, 4) -> (9.5, 7) projected
  point P0 (0, 0)
  dimension "d129" = 0.2
  dimension "d135" = 1
  dimension "d136" = 0.2
  constraints: 1 centre point
  measures "d129" diameter of A0
  measures "d135" distance from line of L0 A0.centre
  measures "d136" distance from line of L1 A0.centre
extrude "Extrusion24" cut sketch "Sketch22" against normal through all
pattern_linear "Rectangular Pattern2" count 4 spacing 2 along (-1, 0, 0) of "Extrusion24"
equation "\"d50\" = d49"
equation "\"d51\" = d49"
equation "\"d52\" = d49"
equation "\"d72\" = d69"
equation "\"d77\" = d76"
equation "\"d81\" = d80"
equation "\"d102\" = d101"
equation "\"d103\" = d101"
body "Solid1"
